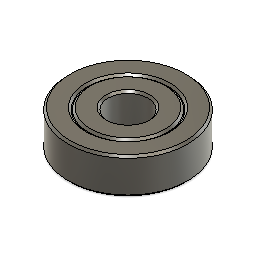
LR2051-821 (Autodesk Fusion 360 design; units mm, degrees)
Autodesk Fusion 360 part; units mm, degrees
sketch "profile" plane through (0, 0, 0) normal (0, 0, 1) x (1, 0, 0) in component "LR2051-821"
  line L0 (0, 0) -> (0, 9) construction
  line L1 (-5, 9) -> (-15, 9)
  line L2 (-15, 9) -> (-15, 0)
  line L3 (-15, 0) -> (-5, 0)
  line L4 (-5, 9) -> (-5, 0)
  line L5 (0, 9) -> (-5, 9) construction
  line L6 (-5, 0) -> (0, 0) construction
  line L7 (-10, 0) -> (-10, 1.5) construction
  line L8 (-10, 1.5) -> (-11.5, 3) construction
  line L9 (-11.5, 3) -> (-8.5, 6) construction
  line L10 (-8.5, 6) -> (-10, 7.5) construction
  line L11 (-10, 7.5) -> (-10, 9) construction
  line L12 (-5, 4.5) -> (-15, 4.5) construction
  line L13 (-10, 7.5) -> (-10, 1.5) construction
  line L14 (-9.9, 0) -> (-9.9, 1.5414)
  line L15 (-9.9, 1.5414) -> (-11.3586, 3)
  line L16 (-11.3586, 3) -> (-8.3586, 6)
  line L17 (-8.3586, 6) -> (-9.9, 7.5414)
  line L18 (-9.9, 7.5414) -> (-9.9, 9)
  line L19 (-10.1, 0) -> (-10.1, 1.4586)
  line L20 (-10.1, 1.4586) -> (-11.6414, 3)
  line L21 (-11.6414, 3) -> (-8.6414, 6)
  line L22 (-8.6414, 6) -> (-10.1, 7.4586)
  line L23 (-10.1, 7.4586) -> (-10.1, 9)
  point P0 (-10, 4.5)
  dimension "d4" = 15
  dimension "d5" = 5
  dimension "d6" = 45
  dimension "d7" = 1.5
  dimension "d8" = 1.5
  dimension "d9" = 9
  dimension "d10" = 0.1
  dimension "d11" = -0.1
  constraint coincident L0.start L6.end
  constraint vertical L0
  constraint perpendicular L0 L1
  constraint perpendicular L1 L2
  constraint perpendicular L0 L3
  constraint perpendicular L3 L4
  constraint perpendicular L0 L5
  constraint perpendicular L0 L6
  constraint midpoint L3 L7.start
  constraint perpendicular L3 L7
  constraint midpoint L1 L11.end
  constraint perpendicular L1 L11
  constraint midpoint L4 L12.start
  constraint midpoint L2 L12.end
  constraint parallel L8 L10
  constraint perpendicular L8 L9
  constraint midpoint L12 P0
  constraint coincident L9 P0
  measures "d4" distance of L2 L0.start
  measures "d5" distance of L0.start L4
  measures "d6" angle of L8 L13
  measures "d7" distance of L9.end L13
  measures "d8" distance of L8.end L11
  measures "d9" distance of L1.end L2.end
revolve "Revolve1" add sketch "profile" angle 360 about axis through (0, 0, 0) along (0, 1, 0) contours L1 L3 L4 L14 L15 L16 L17 L18 makes body 1 in component "Inner Shell"
revolve "Revolve1'" add sketch "profile" angle 360 about axis through (0, 0, 0) along (0, 1, 0) separate body contours L1 L2 L3 L19 L20 L21 L22 L23 makes body 2 in component "Outer Shell"
chamfer "Chamfer1" distance 0.5 angle 45 2 edges at (-9.23, 9, 3.58) (-9.23, 0, 3.58) on bodies 1 in component "Inner Shell"
chamfer "Chamfer2" distance 0.5 angle 45 2 edges at (-4.6616, 9, 1.8081) (-4.6616, 0, 1.8081) on bodies 1 in component "Inner Shell"
chamfer "Chamfer1'" distance 0.5 angle 45 2 edges at (-9.4165, 9, 3.6523) (-9.4165, 0, 3.6523) on bodies 2 in component "Outer Shell"
chamfer "Chamfer2'" distance 0.5 angle 45 2 edges at (-13.9849, 9, 5.4242) (-13.9849, 0, 5.4242) on bodies 2 in component "Outer Shell"
fillet "Fillet1" radius 0.5 2 edges at (-7.7929, 6, 3.0226) (-10.5899, 3, 4.1074) on bodies 1 in component "Inner Shell"
fillet "Fillet1'" radius 0.5 2 edges at (-8.0566, 6, 3.1249) (-10.8536, 3, 4.2097) on bodies 2 in component "Outer Shell"
component "LR2051-821" placed x (1, 0, 0) y (0, 1, 0) z (0, 0, 1) at (0, 0, 0)
component "Inner Shell" placed x (1, 0, 0) y (0, 1, 0) z (0, 0, 1) at (0, 0, 0) in component "LR2051-821"
component "Outer Shell" placed x (1, 0, 0) y (0, 1, 0) z (0, 0, 1) at (0, 0, 0) in component "LR2051-821"
equation "inner_dia = 10 mm"
equation "outer_dia = 30 mm"
equation "width = 9 mm"
equation "d4 = outer_dia / 2"
equation "d5 = inner_dia / 2"
equation "d8 = d7"
equation "d9 = width"
equation "d10 = gap / 2"
equation "d11 = -gap / 2"
equation "gap = 0.2 mm"
equation "outer_chamfer = 0.5 mm"
equation "inner_chamfer = 0.5 mm"
equation "d17 = inner_chamfer"
equation "d18 = outer_chamfer"
equation "d19 = inner_chamfer"
equation "d20 = outer_chamfer"
named bodies: "inner_shell", "outer_shell"
